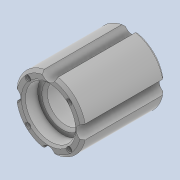
# Autodesk Inventor part: centrifugetool_5mm_tubecollar_v2
Saved by Autodesk Inventor 2021.2 (Build 252289000, 289)
## iProperties
Created: 2021-10-07
Part Number: centrifugetool_5mm_tubecollar_v2
Material: Generic
Document SubType Name: Modeling
Designer: to172
Density: 1 g/cm^3
Appearance: Smooth - Medium Gray
Author: to172
Autodesk Inventor part; units mm, degrees
ref_plane "YZ Plane" through (0, 0, 0) normal (1, 0, 0) x (0, 1, 0)
ref_plane "XZ Plane" through (0, 0, 0) normal (0, 1, 0) x (-1, 0, 0)
sketch "Sketch1" plane through (0, 0, 0) normal (0, 0, 1) x (1, 0, 0)
  circle A0 centre (0, 0) radius 12.5
  circle A1 centre (0, 0) radius 6.6
  circle A2 centre (0, 12.5) radius 2.5
  line L0 (0, 0) -> (0, 15.8185) construction
  circle A3 centre (-12.5, 0) radius 2.5
  circle A4 centre (0, -12.5) radius 2.5
  circle A5 centre (12.5, 0) radius 2.5
  point P0 (12.25, -2.4875)
  point P1 (12.25, 2.4875)
  point P2 (2.4875, 12.25)
  point P3 (-2.4875, 12.25)
  point P4 (-12.25, 2.4875)
  point P5 (-12.25, -2.4875)
  point P6 (-2.4875, -12.25)
  point P7 (2.4875, -12.25)
  dimension "d0" = 25
  dimension "d1" = 13.2
  dimension "d2" = 5
  dimension "d5" = 360
  constraints: 5 centre point, 2 coincident, 2 end point, 1 point on line, 1 vertical, 12 other
  measures "d1" diameter of A1
  measures "d2" diameter of A2
extrude "Extrusion1" add sketch "Sketch1" along normal blind 30 contours A5 A0 A4 A3 A2
chamfer "Chamfer1" distance 1 angle 45 8 edges at (8.8388, -8.8388, 0) (-8.8388, -8.8388, 0) (-8.8388, 8.8388, 0) (8.8388, 8.8388, 0) (8.8388, 8.8388, 30) (8.8388, -8.8388, 30) (-8.8388, -8.8388, 30) (-8.8388, 8.8388, 30)
sketch "Sketch2" plane through (0, 0, 0) normal (0, 0, -1) x (-1, 0, 0)
  circle A0 centre (0, 0) radius 9.075
  dimension "d12" = 18.15
  constraints: 1 centre point, 1 coincident
  measures "d12" diameter of A0
extrude "Extrusion2" cut sketch "Sketch2" against normal blind 5.2
chamfer "Chamfer2" distance 1 angle 45 1 edges at (-6.6, 0, 5.2)
ref_plane "Work Plane1" through (0, 0, 15) normal (0, 0, 1) x (1, 0, 0)
mirror "Mirror1" about plane through (0, 0, 15) normal (0, 0, 1) of "Extrusion2", "Chamfer2"
chamfer "Chamfer3" distance 0.75 angle 45 2 edges at (9.075, 0, 30) (9.075, 0, 0)
sketch "Sketch4" plane through (0, 0, 0) normal (0, 0, -1) x (-1, 0, 0)
  circle A0 centre (0, 0) radius 10.5 construction
  line L0 (0, 0) -> (0, -16.6213) construction
  line L1 (0, 0) -> (-21.5739, 0) construction
  line L2 (0, 0) -> (-13.6342, -13.6342) construction
  circle A1 centre (-7.4246, -7.4246) radius 0.8
  line L3 (0, 0) -> (0, -21.5739) construction
  circle A2 centre (7.4246, -7.4246) radius 0.8
  line L4 (0, 0) -> (21.5739, 0) construction
  circle A3 centre (7.4246, 7.4246) radius 0.8
  line L5 (0, 0) -> (0, 21.5739) construction
  circle A4 centre (-7.4246, 7.4246) radius 0.8
  dimension "d23" = 21
  dimension "d24" = 45
  dimension "d25" = 1.6
  dimension "d28" = 360
  constraints: 12 end point, 4 centre point, 1 coincident, 1 horizontal, 1 point on line, 1 vertical, 24 other
  measures "d24" angle of L0 L2
  measures "d25" diameter of A1
extrude "Extrusion3" cut sketch "Sketch4" against normal blind 2
chamfer "Chamfer4" distance 0.25 angle 45 8 edges at (-7.329, 8.2189, 0) (-7.9186, 6.7954, 0) (8.0539, 7.9186, 0) (6.6304, 7.329, 0) (6.6304, -7.329, 0) (8.0539, -7.9186, 0) (-7.9186, -6.7954, 0) (-7.329, -8.2189, 0)
mirror "Mirror2" about plane through (0, 0, 15) normal (0, 0, 1) of "Extrusion3"
chamfer "Chamfer5" distance 0.25 angle 45 8 edges at (8.0539, 7.9186, 30) (6.6304, 7.329, 30) (6.6304, -7.329, 30) (8.0539, -7.9186, 30) (-7.9186, -6.7954, 30) (-7.329, -8.2189, 30) (-7.329, 8.2189, 30) (-7.9186, 6.7954, 30)
body "Solid1"
